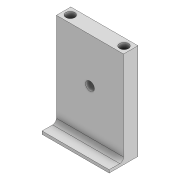
# Autodesk Inventor part: antenna_mast_mount
Saved by Autodesk Inventor 2022 (Build 260153000, 153)
## iProperties
Created: 2022-07-20
Part Number: antenna_mast_mount
Material: Generic
Document SubType Name: Modeling
Designer: Thomas
Density: 1 g/cm^3
Appearance: Default
Author: Thomas
Autodesk Inventor part; units mm, degrees
ref_plane "YZ Plane" through (0, 0, 0) normal (1, 0, 0) x (0, 1, 0)
ref_plane "XZ Plane" through (0, 0, 0) normal (0, 1, 0) x (-1, 0, 0)
ref_plane "XY Plane" through (0, 0, 0) normal (0, 0, 1) x (1, 0, 0)
sketch "Sketch1" plane through (0, 0, 0) normal (0, 0, 1) x (1, 0, 0)
  line L0 (0, 0) -> (70, 0)
  line L1 (70, 0) -> (70, 100)
  line L2 (70, 100) -> (0, 100)
  line L3 (0, 100) -> (0, 0)
  dimension "d0" = 70
  dimension "d1" = 100
  constraints: 8 end point, 2 parallel, 1 horizontal, 1 perpendicular
  measures "d0" distance of L2.end L1.end
  measures "d1" distance of L1.end L0.end
extrude "Extrusion1" add sketch "Sketch1" along normal blind 15
sketch "Sketch3" plane through (0, 100, 0) normal (0, 1, 0) x (1, 0, 0)
  line L0 (0, 0) -> (0, -15) projected
  line L1 (0, -7.5) -> (70, -7.5) construction
  line L2 (70, 0) -> (70, -15) projected
  circle A0 centre (7, -7.5) radius 4.65
  circle A1 centre (63, -7.5) radius 4.65
  dimension "d7" = 9.3
  dimension "d8" = 9.3
  dimension "d9" = 56
  dimension "d10" = 70
  dimension "d11" = 7
  constraints: 2 centre point, 2 end point, 2 midpoint, 2 point on line
  measures "d7" diameter of A0
  measures "d8" diameter of A1
  measures "d9" distance of A1.centre A0.centre
  measures "d10" distance between parallel lines of L0 L2
  measures "d11" distance from line of L0 A0.centre
extrude "Extrusion3" cut sketch "Sketch3" against normal blind 15
sketch "Sketch4" plane through (0, 0, 15) normal (0, 0, 1) x (1, 0, 0)
  line L0 (70, 0) -> (70, 100) projected
  line L1 (0, 0) -> (70, 0)
  line L2 (70, 0) -> (70, 3)
  line L3 (70, 3) -> (0, 3)
  line L4 (0, 3) -> (0, 0)
  dimension "d14" = 3
  constraints: 8 end point, 2 parallel, 1 horizontal, 1 perpendicular, 1 point on line
  measures "d14" distance between parallel lines of L3 L1
extrude "Extrusion4" add sketch "Sketch4" along normal blind 15
fillet "Fillet1" radius 4 1 edges at (35, 3, 15)
sketch "Sketch5" plane through (0, 0, 15) normal (0, 0, 1) x (1, 0, 0)
  line L0 (70, 0) -> (70, 100) projected
  line L1 (0, 0) -> (70, 0) projected
  line L2 (0, 100) -> (0, 0) projected
  line L3 (70, 100) -> (0, 100) projected
  circle A0 centre (35, 53.5) radius 4.625
  line L4 (70, 100) -> (0, 100) projected
  line L5 (35, 100) -> (35, 0)
  line L6 (0, 0) -> (70, 0) projected
  line L7 (70, 7) -> (70, 100) projected
  line L8 (70, 53.5) -> (0, 53.5)
  line L9 (0, 100) -> (0, 7) projected
  dimension "d18" = 9.25
  constraints: 5 midpoint, 4 end point, 1 centre point, 1 coincident
  measures "d18" diameter of A0
sketch "Sketch5 outline for Extrusion5" plane through (0, 0, 15) normal (0, 0, 1) x (1, 0, 0)
  circle A0 centre (35, 53.5) radius 4.625
extrude "Extrusion5" cut sketch "Sketch5 outline for Extrusion5" against normal blind 11 draft -2
equation "\"d8\" = d7"
equation "\"d11\" = -0.5 * d9 + 0.5 * d10"
body "Solid1"
